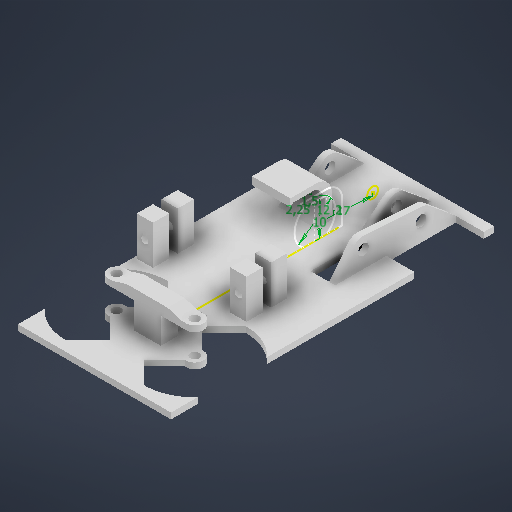
# Autodesk Inventor part: Рама
Saved by Autodesk Inventor 2026.2 (Build 302298000, 298)
## iProperties
Created: 2026-02-19
Part Number: Рама
Material: Типовые
Document SubType Name: Modeling
Designer: Leonid
Density: 1 g/cm^3
Appearance: По умолчанию
Author: Leonid
Autodesk Inventor part; units mm, degrees
ref_plane "YZ Plane" through (0, 0, 0) normal (1, 0, 0) x (0, 1, 0)
ref_plane "XZ Plane" through (0, 0, 0) normal (0, 1, 0) x (-1, 0, 0)
ref_plane "XY Plane" through (0, 0, 0) normal (0, 0, 1) x (1, 0, 0)
sketch "Эскиз1" plane through (0, 0, 0) normal (0, 1, 0) x (-1, 0, 0)
  line L0 (-22.5, -47.5) -> (22.5, -47.5)
  line L1 (22.5, -47.5) -> (22.5, 14.5)
  line L2 (22.5, 47.5) -> (-22.5, 47.5)
  line L3 (-22.5, 47.5) -> (-22.5, 44.5)
  line L4 (-22.5, -47.5) -> (22.5, 47.5) construction
  line L5 (22.5, -47.5) -> (-22.5, 47.5) construction
  line L6 (22.5, 29.5) -> (-22.5, 29.5) construction
  line L7 (-22.5, 44.5) -> (-22.5, 14.5)
  line L8 (-22.5, 14.5) -> (-22.5, -47.5)
  line L9 (22.5, 14.5) -> (22.5, 44.5)
  line L10 (22.5, 44.5) -> (22.5, 47.5)
  circle A0 centre (11.5, 29.5) radius 1.325
  line L11 (22.5, 44.5) -> (5, 44.5)
  line L12 (-22.5, 44.5) -> (-5, 44.5)
  arc A1 (11.5, 27) -> (11.5, 32) centre (11.5, 29.5) ccw
  line L13 (11.5, 32) -> (5, 32)
  circle A2 centre (-11.5, 29.5) radius 1.325
  arc A3 (-11.5, 32) -> (-11.5, 27) centre (-11.5, 29.5) ccw
  line L14 (-11.5, 32) -> (-5, 32)
  line L15 (11.5, 27) -> (-11.5, 27)
  line L16 (22.5, 14.5) -> (-22.5, 14.5)
  line L17 (5, 32) -> (5, 44.5)
  line L18 (-5, 32) -> (-5, 44.5)
  line L19 (-11.5, 44.5) -> (-5, 38)
  line L20 (-11.5, 44.5) -> (-2.3076, 44.5) construction
  line L21 (11.5, 44.5) -> (5, 38)
  line L22 (11.5, 44.5) -> (20.6924, 44.5) construction
  line L23 (5, 38) -> (11, 32)
  line L24 (-5, 38) -> (-11, 32)
  arc A4 (-11.5, 44.5) -> (-22.5, 39.698) centre (-11.5, 29.5) ccw
  arc A5 (22.5, 39.698) -> (11.5, 44.5) centre (11.5, 29.5) ccw
  arc A6 (-22.5, 19.302) -> (-11.5, 14.5) centre (-11.5, 29.5) ccw
  arc A7 (11.5, 14.5) -> (22.5, 19.302) centre (11.5, 29.5) ccw
  line L25 (-11.5, 44.5) -> (-11.5, 14.5) construction
  line L26 (11.5, 44.5) -> (11.5, 14.5) construction
  line L27 (-11, 27) -> (-5, 21)
  line L28 (-11, 27) -> (-2.5147, 27) construction
  line L29 (-5, 21) -> (-11.5, 14.5)
  line L30 (11.5, 14.5) -> (5, 21)
  line L31 (11.5, 14.5) -> (20.6924, 14.5) construction
  line L32 (5, 21) -> (11, 27)
  line L33 (-5.75, 8.55) -> (-10.5, 8.55)
  line L34 (-10.5, 8.55) -> (-10.5, 13.3)
  line L35 (-10.5, 13.3) -> (-5.75, 13.3)
  line L36 (-5.75, 13.3) -> (-5.75, 8.55)
  line L37 (17, 8.55) -> (21.75, 8.55)
  line L38 (21.75, 8.55) -> (21.75, 13.3)
  line L39 (21.75, 13.3) -> (17, 13.3)
  line L40 (17, 13.3) -> (17, 8.55)
  line L41 (-5.75, 1.3) -> (-10.5, 1.3)
  line L42 (-10.5, 1.3) -> (-10.5, 6.05)
  line L43 (-10.5, 6.05) -> (-5.75, 6.05)
  line L44 (-5.75, 6.05) -> (-5.75, 1.3)
  line L45 (17, 1.3) -> (21.75, 1.3)
  line L46 (21.75, 1.3) -> (21.75, 6.05)
  line L47 (21.75, 6.05) -> (17, 6.05)
  line L48 (17, 6.05) -> (17, 1.3)
  line L49 (22.5, -44.5) -> (-22.5, -44.5)
  line L50 (-22.5, -24.104) -> (-14.25, -24.104)
  line L51 (-14.25, -24.104) -> (-14.25, -44.5)
  line L52 (22.5, -24.104) -> (14.25, -24.104)
  line L53 (14.25, -24.104) -> (14.25, -44.5)
  line L54 (-12.5, -25.63) -> (-7, -25.63)
  line L55 (-7, -25.63) -> (-7, -42.974)
  line L56 (-7, -42.974) -> (-12.5, -42.974)
  line L57 (-12.5, -42.974) -> (-12.5, -25.63)
  line L58 (-12.5, -34.302) -> (-14.25, -34.302) construction
  line L59 (-4, 27) -> (4, 27)
  line L60 (4, 27) -> (4, 32)
  line L61 (4, 32) -> (-4, 32)
  line L62 (-4, 32) -> (-4, 27)
  line L63 (-4, 27) -> (4, 32) construction
  line L64 (4, 27) -> (-4, 32) construction
  line L65 (-7, -25.63) -> (-12.5, -25.63)
  line L66 (-12.5, -25.63) -> (-12.5, -9.052)
  line L67 (-12.5, -9.052) -> (-7, -9.052)
  line L68 (-7, -9.052) -> (-7, -25.63)
  point P0 (0, 0)
  point P1 (13.75, 44.5)
  point P2 (-12.5, -44.5)
  point P3 (0, 29.5)
  point P4 (-4, 27)
  point P5 (4, 27)
  point P6 (-7, -17.341)
  dimension "d0" = 45
  dimension "d6" = 3
  dimension "d7" = 2.65
  dimension "d8" = 11
  dimension "d14" = 2.65
  dimension "d15" = 11
  dimension "d16" = 2.5
  dimension "d19" = 10
  dimension "d20" = 12.5
  dimension "d22" = 95
  dimension "d23" = 12.5
  dimension "d25" = 23
  dimension "d26" = 45
  dimension "d27" = 135
  dimension "d29" = 23
  dimension "d30" = 45
  dimension "d31" = 135
  dimension "d37" = 0.5
  dimension "d38" = 32.25
  dimension "d39" = 22.75
  dimension "d40" = 4.75
  dimension "d42" = 5.95
  dimension "d43" = 32.25
  dimension "d44" = 22.75
  dimension "d45" = 4.75
  dimension "d46" = 2.5
  dimension "d60" = 20.3961
  dimension "d61" = 3
  dimension "d62" = 20.396
  dimension "d63" = 8.25
  dimension "d71" = 1.75
  dimension "d72" = 5.5
  dimension "d73" = 17.344
  dimension "d120" = 8
  dimension "d129" = 5.5
  dimension "d130" = 0
  dimension "d131" = 6.763
  constraints: 138 end point, 31 point on line, 23 parallel, 23 perpendicular, 17 horizontal, 12 point on circle, 11 equal length, 11 midpoint, 8 centre point, 6 coincident, 6 collinear, 6 tangent, 1 vertical
  measures "d0" distance of L2.end L2.start
  measures "d6" distance of L9.end L2.start
  measures "d7" diameter of A0
  measures "d8" distance from line of A0.centre L9
  measures "d14" diameter of A2
  measures "d15" distance from line of L7 A2.centre
  measures "d16" radius of A3
  measures "d19" distance between parallel lines of L18 L17
  measures "d20" distance between parallel lines of L16 L15
  measures "d22" distance between parallel lines of L0 L2
  measures "d23" vertical distance of L3.end L14.start
  measures "d25" distance of A2.centre A0.centre
  measures "d26" angle of L19 L20
  measures "d27" angle of L21 L22
  measures "d29" distance of L19.start L21.start
  measures "d30" angle of L27 L28
  measures "d31" angle of L31 L30
  measures "d37" distance of L15.start L32.end
  measures "d38" distance between parallel lines of L34 L38
  measures "d39" distance between parallel lines of L36 L40
  measures "d40" distance between parallel lines of L35 L33
  measures "d42" distance from line of L25.end L33
  measures "d43" distance between parallel lines of L42 L46
  measures "d44" distance between parallel lines of L44 L48
  measures "d45" distance between parallel lines of L43 L41
  measures "d46" distance between parallel lines of L33 L43
  measures "d60" distance of A6.start A4.end
  measures "d61" distance between parallel lines of L0 L49
  measures "d62" distance of L49.end L50.start
  measures "d63" distance of L50.start L50.end
  measures "d71" distance between parallel lines of L51 L57
  measures "d72" distance between parallel lines of L57 L55
  measures "d73" distance between parallel lines of L56 L54
  measures "d120" distance between parallel lines of L60 L62
  measures "d129" distance from line of L39.end L1
  measures "d130" distance between parallel lines of L54 L65
  measures "d131" distance from line of L50 point (-7, -17.341)
extrude "Выдавливание1" add sketch "Эскиз1" along normal blind 1.75 contours L8 L49 L1 L0 | L8 L16 L1 L52 L53 L49 L51 L50 | L7 A6 L16 | L16 A7 L9 | L29 L27 L15 L32 L30 L16 | L7 L12 A4 | A5 L11 L9 | L3 L2 L10 L11 L17 L13 A1 L15 L60 L61 L62 A3 L14 L18 L12 | L12 L18 L19 | L21 L17 L11 | L18 L14 L24 | L62 L61 L60 L15 | L23 L13 L17 | L33 L34 L35 L36 | L40 L39 L38 L37 | L41 L42 L43 L44 | L48 L47 L46 L45
extrude "Выдавливание3" add sketch "Эскиз1" along normal blind 13.25 contours L33 L34 L35 L36 | L40 L39 L38 L37 | L41 L42 L43 L44 | L48 L47 L46 L45
sketch "Эскиз3" plane through (10.5, 1.75, 1.3) normal (0, 0, -1) x (-1, 0, 0)
  line L0 (-12, 0) -> (33, 0) projected
  line L1 (0, 0) -> (0, 11.5) projected
  point P0 (10.5, -1.75)
  point P1 (2.375, 5.95)
  point P2 (29.875, 5.95)
  dimension "d49" = 27.5
  dimension "d50" = 5.95
  dimension "d51" = 2.375
  dimension "d52" = 5.95
  measures "d49" distance of point (29.875, 5.95) point (2.375, 5.95)
  measures "d50" distance from line of L0 point (2.375, 5.95)
  measures "d51" distance from line of L1 point (2.375, 5.95)
  measures "d52" distance from line of L0 point (29.875, 5.95)
hole "Отверстие1" at (8.125, 7.7, 1.3) at (-19.375, 7.7, 1.3) direction (0, 0, 1) diameter 2.1 end through all
sketch "Эскиз4" plane through (14.25, 0, -24.104) normal (1, 0, 0) x (0, 0, -1)
  line L0 (0, 1.75) -> (20.396, 1.75) projected
  circle A0 centre (10.198, 5.6) radius 1.575
  line L1 (10.198, 5.6) -> (10.198, 1.75) construction
  arc A1 (12.4201, 8.3041) -> (7.9759, 8.3041) centre (10.198, 5.6) ccw
  line L2 (0, 1.75) -> (7.9759, 8.3041)
  line L3 (12.4201, 8.3041) -> (20.396, 1.75)
  line L4 (18.87, 1.75) -> (-15.052, 1.75) projected
  circle A2 centre (-6.763, 6.75) radius 1.575
  line L5 (0, 0) -> (0, 1.75) projected
  arc A3 (-6.5262, 10.242) -> (-9.5321, 8.8906) centre (-6.763, 6.75) ccw
  line L6 (-15.052, 1.75) -> (-9.5321, 8.8906)
  line L7 (-6.5262, 10.242) -> (12.9523, 8.9213)
  point P0 (-24.104, 0)
  point P1 (10.4348, 9.092)
  dimension "d64" = 3.15
  dimension "d65" = 3.85
  dimension "d66" = 3.5
  dimension "d132" = 3.15
  dimension "d133" = 6.763
  dimension "d134" = 5
  dimension "d135" = 3.5
  constraints: 10 end point, 5 tangent, 4 centre point, 4 point on circle, 2 coincident, 1 midpoint, 1 vertical
  measures "d64" diameter of A0
  measures "d65" distance of L1.start L1.end
  measures "d66" radius of A1
  measures "d132" diameter of A2
  measures "d133" distance from line of L5 A2.centre
  measures "d134" distance from line of L4 A2.centre
  measures "d135" radius of A3
extrude "Выдавливание12" add sketch "Эскиз1" along normal blind 9.45 contours L62 L61 L60 L15
ref_plane "РабПлоскость4" through (-22.5, 0, 17.5) normal (0, 0, 1) x (1, 0, 0)
sketch "Эскиз7" plane through (-22.5, 0, 17.5) normal (0, 0, 1) x (1, 0, 0)
  circle A0 centre (22.5, 8) radius 7
  line L0 (0, 1.75) -> (45, 1.75) projected
  line L1 (22.5, 1.75) -> (22.5, 8) construction
  point P0 (22.5, 0)
  point P1 (25.6524, 1.75)
  point P2 (19.3476, 1.75)
  dimension "d110" = 14
  dimension "d111" = 6.25
  constraints: 2 end point, 1 centre point, 1 midpoint, 1 vertical
  measures "d110" diameter of A0
  measures "d111" distance of L1.start L1.end
extrude "Выдавливание15" cut sketch "Эскиз7" along normal blind 9.5 contours L0 A0 picked at (21.9599, 1.5634)
sketch "Эскиз8" plane through (0, 9.45, 0) normal (0, 1, 0) x (1, 0, 0)
  arc A0 (11.5, -32) -> (11.5, -27) centre (11.5, -29.5) ccw projected
  line L0 (-11.5, -27) -> (11.5, -27) projected
  arc A1 (-11.5, -27) -> (-11.5, -32) centre (-11.5, -29.5) ccw projected
  line L1 (-11.5, -32) -> (-11, -32) construction
  line L2 (-11.5, -32) -> (11.5, -32)
  circle A2 centre (-11.5, -29.5) radius 1.325 projected
  circle A3 centre (11.5, -29.5) radius 1.325 projected
  point P0 (0, 0)
  constraints: 2 end point, 1 horizontal, 1 tangent
extrude "Выдавливание16" add sketch "Эскиз8" along normal blind 1.75
sketch "Эскиз9" plane through (-4, 1.75, 32) normal (0, 0, 1) x (1, 0, 0)
  line L0 (-8.825, 9.45) -> (-6.175, 9.45) projected
  line L1 (14.175, 9.45) -> (16.825, 9.45) projected
  line L2 (-6.175, 9.45) -> (-2, 10.7)
  line L3 (14.175, 9.45) -> (10, 10.7)
  line L4 (-7.5, 9.45) -> (15.5, 9.45) projected
  line L5 (-2, 10.7) -> (2, 10.7)
  line L6 (6, 10.7) -> (10, 10.7)
  line L7 (0, 7.7) -> (-7.5, 7.7) projected
  line L8 (0, 10.7) -> (0, 7.7) construction
  line L9 (2, 10.7) -> (6, 10.7)
  point P0 (4, -1.75)
  dimension "d125" = 1.25
  dimension "d126" = 4
  constraints: 12 end point, 2 collinear, 2 equal length, 1 midpoint, 1 vertical
  measures "d125" distance between parallel lines of L4 L6
  measures "d126" distance of L6.start L3.end
extrude "Выдавливание17" add sketch "Эскиз9" against normal blind 5
extrude "Выдавливание18" add sketch "Эскиз4" against normal blind 9 contours L2 A1 L3 L0
extrude "Выдавливание19" cut sketch "Эскиз4" against normal blind 7.25 contours L2 A1 L3 L0
extrude "Выдавливание20" add sketch "Эскиз4" against normal blind 1.75 contours L2 A1 L3 L0
mirror "Зеркальное отражение2" about plane through (0, 0, 0) normal (1, 0, 0) of "Выдавливание20"
extrude "Выдавливание21" add sketch "Эскиз4" against normal blind 1.75 contours L4 L6 A3 L7 A1 L2
sketch "Эскиз11" plane through (0, 0, 0) normal (1, 0, 0) x (0, 1, 0)
  arc A0 (11.75, -14.0243) -> (1.75, -14.0243) centre (6.75, -17.3409) ccw
  line L0 (11.75, -14.0243) -> (11.75, -20.6576)
  line L1 (11.75, -17.3409) -> (1.75, -17.3409) construction
  line L2 (1.75, -14.0243) -> (1.75, -20.6576)
  line L3 (1.75, -9.052) -> (1.75, -24.104) construction
  circle A1 centre (5.6, -34.302) radius 1.575 projected
  line L4 (1.75, 19.302) -> (1.75, -24.104) projected
  line L5 (13.25, -13.1057) -> (13.25, -20.6576)
  arc A2 (1.75, -14.0243) -> (1.75, -20.6576) centre (6.75, -17.3409) ccw construction
  arc A3 (1.75, -20.6576) -> (11.75, -20.6576) centre (6.75, -17.3409) ccw
  line L6 (8.5666, -25.3409) -> (1.75, -25.3409)
  line L7 (0, -44.5) -> (0, -24.104) projected
  line L8 (1.75, -25.3409) -> (1.75, -20.6576)
  arc A4 (8.5666, -25.3409) -> (13.25, -20.6576) centre (8.5666, -20.6576) ccw
  line L9 (11.75, -20.6576) -> (8.5666, -20.6576) construction
  line L10 (13.25, -13.1057) -> (11, -13.1057)
  point P0 (0, 0)
  point P1 (6.75, -23.3409)
  point P2 (1.75, -24.104)
  dimension "d144" = 12
  dimension "d145" = 10
  dimension "d147" = 17
  dimension "d149" = 1.5
  dimension "d150" = 2
  dimension "d152" = 2.25
  constraints: 16 end point, 11 point on circle, 4 centre point, 3 horizontal, 3 midpoint, 2 perpendicular, 2 tangent, 1 coincident, 1 collinear, 1 point on line, 1 vertical
  measures "d144" diameter of A0
  measures "d145" distance of L1.start L1.end
  measures "d147" distance of A0.centre A1.centre
  measures "d149" distance between parallel lines of L5 L0
  measures "d150" distance from line of point (6.75, -23.341) L6
  measures "d152" distance of L5.start L10.end
extrude "Выдавливание22" add sketch "Эскиз11" against normal blind 14.25 contours A0 L10 L5 A4 L6 L8 L4 A3 L0
extrude "Выдавливание23" cut sketch "Эскиз11" against normal blind 3 contours A0 L10 L5 A4 L6 L8 L4 A3 L0
